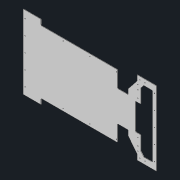
# Autodesk Inventor part: bellypanKJversion
Saved by Autodesk Inventor 2022 (Build 260153000, 153)
## iProperties
Created: 2022-09-22
Part Number: bellypanKJversion
Material: Generic
Document SubType Name: Modeling
Designer: Kieran Jarvis
Density: 1 g/cm^3
Appearance: Default
Author: Kieran Jarvis
Autodesk Inventor part; units mm, degrees
ref_plane "YZ Plane" through (0, 0, 0) normal (1, 0, 0) x (0, 1, 0)
ref_plane "XZ Plane" through (0, 0, 0) normal (0, 1, 0) x (-1, 0, 0)
ref_plane "XY Plane" through (0, 0, 0) normal (0, 0, 1) x (1, 0, 0)
sketch "Sketch1" plane through (0, 0, 0) normal (0, 0, 1) x (1, 0, 0)
  line L0 (0, 0) -> (0, 600) projected
  line L1 (900, 0) -> (900, 600) projected
  circle A0 centre (630, 497.5) radius 2.5 projected
  circle A1 centre (630, 102.5) radius 2.5 projected
  circle A2 centre (450, 102.5) radius 2.5 projected
  circle A3 centre (270, 102.5) radius 2.5 projected
  circle A4 centre (270, 497.5) radius 2.5 projected
  circle A5 centre (450, 497.5) radius 2.5 projected
  circle A6 centre (887.5, 500) radius 2.5 projected
  circle A7 centre (887.5, 400) radius 2.5 projected
  circle A8 centre (887.5, 300) radius 2.5 projected
  circle A9 centre (887.5, 200) radius 2.5 projected
  circle A10 centre (887.5, 100) radius 2.5 projected
  circle A11 centre (12.5, 500) radius 2.5 projected
  circle A12 centre (12.5, 400) radius 2.5 projected
  circle A13 centre (12.5, 300) radius 2.5 projected
  circle A14 centre (12.5, 200) radius 2.5 projected
  circle A15 centre (12.5, 100) radius 2.5 projected
  line L2 (875, 550) -> (25, 550) projected
  line L3 (875, 50) -> (25, 50) projected
  line L4 (875, 550) -> (900, 550)
  line L5 (875, 50) -> (900, 50)
  line L6 (25, 550) -> (0, 550)
  line L7 (25, 50) -> (0, 50)
  line L8 (875, 0) -> (875, 600) construction
  line L9 (795, 510) -> (795, 90) construction
  line L10 (875, 510) -> (25, 510) construction
  line L11 (875, 90) -> (25, 90) construction
  line L12 (875, 510) -> (875, 90)
  line L13 (875, 90) -> (815, 90)
  line L14 (815, 90) -> (815, 115)
  line L15 (815, 115) -> (795, 115)
  line L16 (875, 510) -> (815, 510)
  line L17 (815, 510) -> (815, 485)
  line L18 (815, 485) -> (795, 485)
  line L19 (763, 390) -> (787, 390) construction
  line L20 (787, 210) -> (763, 210) construction
  line L21 (795, 485) -> (795, 390)
  line L22 (758, 510) -> (758, 385) construction
  line L23 (758, 215) -> (758, 90) construction
  line L24 (795, 390) -> (758, 390)
  line L25 (795, 115) -> (795, 210)
  line L26 (795, 210) -> (758, 210)
  line L27 (758, 390) -> (758, 210)
  line L28 (780, 53) -> (780, 87) construction
  line L29 (780, 547) -> (780, 513) construction
  line L30 (780, 50) -> (770, 50) construction
  line L31 (770, 50) -> (770, 90) construction
  line L32 (770, 90) -> (780, 90) construction
  line L33 (780, 90) -> (780, 50) construction
  line L34 (780, 87) -> (120, 87) construction
  line L35 (780, 513) -> (120, 513) construction
  line L36 (770, 50) -> (770, 87)
  line L37 (770, 87) -> (120, 87)
  line L38 (120, 87) -> (120, 53) construction
  line L39 (120, 87) -> (120, 50)
  line L40 (780, 550) -> (770, 550) construction
  line L41 (770, 550) -> (770, 513) construction
  line L42 (770, 513) -> (780, 513) construction
  line L43 (780, 513) -> (780, 550) construction
  line L44 (770, 550) -> (770, 513)
  line L45 (770, 513) -> (120, 513)
  line L46 (120, 513) -> (120, 550)
  line L47 (795, 115) -> (815, 90)
  line L48 (815, 510) -> (795, 485)
  circle A16 centre (823.5, 530) radius 3 projected
  circle A17 centre (788.5, 530) radius 3 projected
  circle A18 centre (823.5, 70) radius 3 projected
  circle A19 centre (788.5, 70) radius 3 projected
  circle A20 centre (823.5, 70) radius 2.5
  circle A21 centre (788.5, 70) radius 2.5
  circle A22 centre (823.5, 530) radius 2.5
  circle A23 centre (788.5, 530) radius 2.5
  dimension "d0" = 60
  dimension "d1" = 25
  dimension "d2" = 60
  dimension "d3" = 25
  dimension "d4" = 10
  dimension "d5" = 10
  dimension "d37" = 5
  dimension "d38" = 5
  dimension "d39" = 5
  constraints: 64 end point, 29 point on line, 8 perpendicular, 6 parallel, 4 centre point, 4 coincident, 2 collinear, 2 horizontal, 2 vertical, 1 equal radius
  measures "d0" distance of L11.start L13.end
  measures "d1" distance of L13.end L14.end
  measures "d2" distance of L10.start L16.end
  measures "d3" distance of L16.end L17.end
  measures "d4" distance of L31.end L32.end
  measures "d5" distance of L42.end L41.end
  measures "d37" diameter of A20
  measures "d38" diameter of A22
  measures "d39" diameter of A23
extrude "Extrusion1" add sketch "Sketch1" along normal blind 3 contours L0 L6 L2 L46 L45 L44 L4 L1 L5 L3 L36 L37 L39 L7 | A16 | A17 | A18 | A19
fillet "Fillet1" radius 5 14 edges at (875, 90, 1.5) (815, 90, 1.5) (795, 115, 1.5) (795, 210, 1.5) (758, 210, 1.5) (758, 390, 1.5) (795, 390, 1.5) (795, 485, 1.5) (815, 510, 1.5) (875, 510, 1.5) (770, 87, 1.5) (120, 87, 1.5) (120, 513, 1.5) (770, 513, 1.5)
sketch "Sketch2" plane through (0, 0, 0) normal (0, 0, -1) x (-1, 0, 0)
  circle A0 centre (-12.5, 100) radius 2.5 projected
  circle A1 centre (-12.5, 300) radius 2.5 projected
  circle A2 centre (-12.5, 500) radius 2.5 projected
  circle A3 centre (-887.5, 200) radius 2.5 projected
  circle A4 centre (-887.5, 400) radius 2.5 projected
  circle A5 centre (-450, 497.5) radius 2.5 projected
  circle A6 centre (-270, 497.5) radius 2.5 projected
  circle A7 centre (-270, 102.5) radius 2.5 projected
  circle A8 centre (-450, 102.5) radius 2.5 projected
  circle A9 centre (-630, 102.5) radius 2.5 projected
  circle A10 centre (-630, 497.5) radius 2.5 projected
  circle A11 centre (-887.5, 500) radius 2.5 projected
  circle A12 centre (-887.5, 300) radius 2.5 projected
  circle A13 centre (-887.5, 100) radius 2.5 projected
  circle A14 centre (-12.5, 400) radius 2.5 projected
  circle A15 centre (-12.5, 200) radius 2.5 projected
  arc A16 (-765, 87) -> (-770, 82) centre (-765, 82) ccw projected
  line L0 (-125, 87) -> (-765, 87) projected
  arc A17 (-120, 82) -> (-125, 87) centre (-125, 82) ccw projected
  line L1 (-120, 50) -> (-120, 82) projected
  line L2 (0, 50) -> (-120, 50) projected
  line L3 (0, 550) -> (0, 50) projected
  line L4 (-120, 550) -> (0, 550) projected
  line L5 (-120, 518) -> (-120, 550) projected
  arc A18 (-125, 513) -> (-120, 518) centre (-125, 518) ccw projected
  line L6 (-765, 513) -> (-125, 513) projected
  arc A19 (-770, 518) -> (-765, 513) centre (-765, 518) ccw projected
  line L7 (-770, 550) -> (-770, 518) projected
  line L8 (-900, 550) -> (-770, 550) projected
  line L9 (-900, 50) -> (-900, 550) projected
  line L10 (-770, 50) -> (-900, 50) projected
  line L11 (-770, 82) -> (-770, 50) projected
  arc A20 (-795, 395) -> (-790, 390) centre (-790, 395) ccw projected
  line L12 (-763, 390) -> (-790, 390) projected
  arc A21 (-758, 385) -> (-763, 390) centre (-763, 385) ccw projected
  line L13 (-758, 215) -> (-758, 385) projected
  arc A22 (-763, 210) -> (-758, 215) centre (-763, 215) ccw projected
  line L14 (-790, 210) -> (-763, 210) projected
  arc A23 (-790, 210) -> (-795, 205) centre (-790, 205) ccw projected
  line L15 (-795, 116.7539) -> (-795, 205) projected
  arc A24 (-796.0957, 113.6304) -> (-795, 116.7539) centre (-800, 116.7539) ccw projected
  line L16 (-813.4988, 91.8765) -> (-796.0957, 113.6304) projected
  arc A25 (-817.4031, 90) -> (-813.4988, 91.8765) centre (-817.4031, 95) ccw projected
  line L17 (-870, 90) -> (-817.4031, 90) projected
  arc A26 (-875, 95) -> (-870, 90) centre (-870, 95) ccw projected
  line L18 (-875, 505) -> (-875, 95) projected
  arc A27 (-870, 510) -> (-875, 505) centre (-870, 505) ccw projected
  line L19 (-817.4031, 510) -> (-870, 510) projected
  arc A28 (-813.4988, 508.1235) -> (-817.4031, 510) centre (-817.4031, 505) ccw projected
  line L20 (-796.0957, 486.3696) -> (-813.4988, 508.1235) projected
  arc A29 (-795, 483.2461) -> (-796.0957, 486.3696) centre (-800, 483.2461) ccw projected
  line L21 (-795, 395) -> (-795, 483.2461) projected
  line L22 (-125, 87) -> (-765, 87) construction
  line L23 (-770, 50) -> (-735, 50) construction
  line L24 (-735, 50) -> (-735, 87) construction
  line L25 (-735, 87) -> (-770, 87) construction
  line L26 (-770, 87) -> (-770, 50) construction
  line L27 (-735, 50) -> (-637, 50) construction
  line L28 (-637, 50) -> (-637, 87) construction
  line L29 (-637, 87) -> (-735, 87) construction
  line L30 (-735, 87) -> (-735, 50) construction
  line L31 (-735, 87) -> (-735, 122)
  line L32 (-735, 122) -> (-710, 122)
  line L33 (-710, 122) -> (-710, 197)
  line L34 (-637, 87) -> (-637, 197)
  line L35 (-637, 197) -> (-710, 197)
  line L36 (-758, 215) -> (-758, 385) construction
  line L37 (-758, 300) -> (0, 300) construction
  line L38 (0, 550) -> (0, 50) construction
  line L39 (-735, 513) -> (-735, 478)
  line L40 (-735, 478) -> (-710, 478)
  line L41 (-710, 478) -> (-710, 403)
  line L42 (-637, 513) -> (-637, 403)
  line L43 (-637, 403) -> (-710, 403)
  point P0 (0, 0)
  point P1 (-637, 513)
  point P2 (-735, 513)
  point P3 (-735, 87)
  point P4 (-637, 87)
  dimension "d9" = 35
  dimension "d10" = 98
  dimension "d11" = 35
  dimension "d12" = 25
  dimension "d13" = 75
  constraints: 38 end point, 6 symmetric about line, 5 perpendicular, 4 parallel, 3 point on line, 2 horizontal, 2 midpoint, 1 vertical
  measures "d9" distance of L25.end L24.end
  measures "d10" distance of L29.end L28.end
  measures "d11" distance of L29.end L31.end
  measures "d12" distance of L31.end L32.end
  measures "d13" distance of L32.end L33.end
extrude "Extrusion2" cut sketch "Sketch2" against normal blind 3 contours L31 L32 L33 L35 L34 L0 | L6 L42 L43 L41 L40 L39
fillet "Fillet2" radius 5 10 edges at (735, 87, 1.5) (735, 122, 1.5) (710, 122, 1.5) (710, 197, 1.5) (637, 197, 1.5) (637, 87, 1.5) (637, 403, 1.5) (710, 403, 1.5) (710, 478, 1.5) (735, 478, 1.5)
sketch "Sketch3" plane through (0, 0, 3) normal (0, 0, 1) x (1, 0, 0)
  arc A0 (715, 478) -> (710, 473) centre (715, 473) ccw projected
  line L0 (710, 473) -> (710, 408) projected
  arc A1 (705, 403) -> (710, 408) centre (705, 408) ccw projected
  line L1 (705, 403) -> (642, 403) projected
  arc A2 (637, 408) -> (642, 403) centre (642, 408) ccw projected
  line L2 (637, 408) -> (637, 513) projected
  line L3 (637, 513) -> (125, 513) projected
  arc A3 (120, 518) -> (125, 513) centre (125, 518) ccw projected
  line L4 (120, 518) -> (120, 550) projected
  line L5 (120, 550) -> (0, 550) projected
  line L6 (0, 550) -> (0, 50) projected
  line L7 (0, 50) -> (120, 50) projected
  line L8 (120, 50) -> (120, 82) projected
  arc A4 (125, 87) -> (120, 82) centre (125, 82) ccw projected
  line L9 (125, 87) -> (632, 87) projected
  arc A5 (632, 87) -> (637, 92) centre (632, 92) ccw projected
  line L10 (637, 92) -> (637, 192) projected
  arc A6 (642, 197) -> (637, 192) centre (642, 192) ccw projected
  line L11 (642, 197) -> (705, 197) projected
  arc A7 (710, 192) -> (705, 197) centre (705, 192) ccw projected
  line L12 (710, 192) -> (710, 127) projected
  arc A8 (710, 127) -> (715, 122) centre (715, 127) ccw projected
  line L13 (715, 122) -> (730, 122) projected
  arc A9 (735, 117) -> (730, 122) centre (730, 117) ccw projected
  line L14 (735, 117) -> (735, 92) projected
  arc A10 (735, 92) -> (740, 87) centre (740, 92) ccw projected
  line L15 (740, 87) -> (765, 87) projected
  arc A11 (770, 82) -> (765, 87) centre (765, 82) ccw projected
  line L16 (770, 82) -> (770, 50) projected
  line L17 (770, 50) -> (900, 50) projected
  line L18 (900, 50) -> (900, 550) projected
  line L19 (900, 550) -> (770, 550) projected
  line L20 (770, 550) -> (770, 518) projected
  arc A12 (765, 513) -> (770, 518) centre (765, 518) ccw projected
  line L21 (765, 513) -> (735, 513) projected
  line L22 (735, 513) -> (735, 483) projected
  arc A13 (730, 478) -> (735, 483) centre (730, 483) ccw projected
  line L23 (730, 478) -> (715, 478) projected
  circle A14 centre (12.5, 200) radius 2.5 projected
  circle A15 centre (12.5, 400) radius 2.5 projected
  circle A16 centre (887.5, 100) radius 2.5 projected
  circle A17 centre (887.5, 300) radius 2.5 projected
  circle A18 centre (887.5, 500) radius 2.5 projected
  circle A19 centre (630, 497.5) radius 2.5 projected
  circle A20 centre (630, 102.5) radius 2.5 projected
  circle A21 centre (450, 102.5) radius 2.5 projected
  circle A22 centre (270, 102.5) radius 2.5 projected
  circle A23 centre (270, 497.5) radius 2.5 projected
  circle A24 centre (450, 497.5) radius 2.5 projected
  circle A25 centre (887.5, 400) radius 2.5 projected
  circle A26 centre (887.5, 200) radius 2.5 projected
  circle A27 centre (12.5, 500) radius 2.5 projected
  circle A28 centre (12.5, 300) radius 2.5 projected
  circle A29 centre (12.5, 100) radius 2.5 projected
  arc A30 (790, 390) -> (795, 395) centre (790, 395) ccw projected
  line L24 (795, 395) -> (795, 483.2461) projected
  arc A31 (796.0957, 486.3696) -> (795, 483.2461) centre (800, 483.2461) ccw projected
  line L25 (796.0957, 486.3696) -> (813.4988, 508.1235) projected
  arc A32 (817.4031, 510) -> (813.4988, 508.1235) centre (817.4031, 505) ccw projected
  line L26 (817.4031, 510) -> (870, 510) projected
  arc A33 (875, 505) -> (870, 510) centre (870, 505) ccw projected
  line L27 (875, 505) -> (875, 95) projected
  arc A34 (870, 90) -> (875, 95) centre (870, 95) ccw projected
  line L28 (870, 90) -> (817.4031, 90) projected
  arc A35 (813.4988, 91.8765) -> (817.4031, 90) centre (817.4031, 95) ccw projected
  line L29 (813.4988, 91.8765) -> (796.0957, 113.6304) projected
  arc A36 (795, 116.7539) -> (796.0957, 113.6304) centre (800, 116.7539) ccw projected
  line L30 (795, 116.7539) -> (795, 205) projected
  arc A37 (795, 205) -> (790, 210) centre (790, 205) ccw projected
  line L31 (790, 210) -> (763, 210) projected
  arc A38 (758, 215) -> (763, 210) centre (763, 215) ccw projected
  line L32 (758, 215) -> (758, 385) projected
  arc A39 (763, 390) -> (758, 385) centre (763, 385) ccw projected
  line L33 (763, 390) -> (790, 390) projected
  line L34 (795, 510) -> (795, 90) projected
  line L35 (763, 390) -> (790, 390) construction
  line L36 (795, 510) -> (775, 510) construction
  line L37 (775, 510) -> (775, 390) construction
  line L38 (775, 390) -> (795, 390) construction
  line L39 (795, 390) -> (795, 510) construction
  line L40 (795, 510) -> (775, 510) construction
  line L41 (775, 510) -> (775, 465) construction
  line L42 (775, 465) -> (795, 465) construction
  line L43 (795, 465) -> (795, 510) construction
  line L44 (795, 510) -> (775, 510) construction
  line L45 (775, 510) -> (775, 495) construction
  line L46 (775, 495) -> (795, 495) construction
  line L47 (795, 495) -> (795, 510) construction
  line L48 (795, 90) -> (775, 90) construction
  line L49 (775, 90) -> (775, 135) construction
  line L50 (775, 135) -> (795, 135) construction
  line L51 (795, 135) -> (795, 90) construction
  line L52 (795, 90) -> (775, 90) construction
  line L53 (775, 90) -> (775, 105) construction
  line L54 (775, 105) -> (795, 105) construction
  line L55 (795, 105) -> (795, 90) construction
  circle A40 centre (775, 105) radius 2.5 projected
  circle A41 centre (775, 135) radius 2.5 projected
  line L56 (775, 135) -> (795.2819, 135) construction
  line L57 (795.2819, 135) -> (795.2819, 185) construction
  line L58 (795.2819, 185) -> (775, 185) construction
  line L59 (775, 185) -> (775, 135) construction
  line L60 (795, 465) -> (775, 465) construction
  line L61 (775, 465) -> (775, 415) construction
  line L62 (775, 415) -> (795, 415) construction
  line L63 (795, 415) -> (795, 465) construction
  point P0 (0, 0)
  dimension "d17" = 20
  dimension "d18" = 45
  dimension "d19" = 15
  dimension "d20" = 20
  dimension "d21" = 45
  dimension "d22" = 20
  dimension "d23" = 15
  dimension "d31" = 50
  dimension "d32" = 50
  constraints: 56 end point, 14 parallel, 7 horizontal, 7 perpendicular, 6 coincident, 4 point on line
  measures "d17" distance of L38.end L37.end
  measures "d18" distance of L41.end L40.end
  measures "d19" distance of L45.end L44.end
  measures "d20" distance of L49.end L50.end
  measures "d21" distance of L48.end L49.end
  measures "d22" distance of L53.end L54.end
  measures "d23" distance of L52.end L53.end
  measures "d31" distance of L57.end L56.end
  measures "d32" distance of L61.end L60.end
hole "Hole1" at (775, 465, 3) at (775, 495, 3) at (775, 135, 3) at (775, 105, 3) at (775, 415, 3) at (775, 185, 3) direction (0, 0, -1) diameter 5 depth 8 tip angle 118
sketch "Sketch4" plane through (0, 0, 3) normal (0, 0, 1) x (1, 0, 0)
  circle A0 centre (775, 415) radius 2.5 projected
  circle A1 centre (775, 135) radius 2.5 projected
  circle A2 centre (775, 465) radius 2.5 projected
  circle A3 centre (775, 495) radius 2.5 projected
  circle A4 centre (775, 105) radius 2.5 projected
  circle A5 centre (775, 185) radius 2.5 projected
  arc A6 (715, 478) -> (710, 473) centre (715, 473) ccw projected
  line L0 (710, 473) -> (710, 408) projected
  arc A7 (705, 403) -> (710, 408) centre (705, 408) ccw projected
  line L1 (705, 403) -> (642, 403) projected
  arc A8 (637, 408) -> (642, 403) centre (642, 408) ccw projected
  line L2 (637, 408) -> (637, 513) projected
  line L3 (637, 513) -> (125, 513) projected
  arc A9 (120, 518) -> (125, 513) centre (125, 518) ccw projected
  line L4 (120, 518) -> (120, 550) projected
  line L5 (120, 550) -> (0, 550) projected
  line L6 (0, 550) -> (0, 50) projected
  line L7 (0, 50) -> (120, 50) projected
  line L8 (120, 50) -> (120, 82) projected
  arc A10 (125, 87) -> (120, 82) centre (125, 82) ccw projected
  line L9 (125, 87) -> (632, 87) projected
  arc A11 (632, 87) -> (637, 92) centre (632, 92) ccw projected
  line L10 (637, 92) -> (637, 192) projected
  arc A12 (642, 197) -> (637, 192) centre (642, 192) ccw projected
  line L11 (642, 197) -> (705, 197) projected
  arc A13 (710, 192) -> (705, 197) centre (705, 192) ccw projected
  line L12 (710, 192) -> (710, 127) projected
  arc A14 (710, 127) -> (715, 122) centre (715, 127) ccw projected
  line L13 (715, 122) -> (730, 122) projected
  arc A15 (735, 117) -> (730, 122) centre (730, 117) ccw projected
  line L14 (735, 117) -> (735, 92) projected
  arc A16 (735, 92) -> (740, 87) centre (740, 92) ccw projected
  line L15 (740, 87) -> (765, 87) projected
  arc A17 (770, 82) -> (765, 87) centre (765, 82) ccw projected
  line L16 (770, 82) -> (770, 50) projected
  line L17 (770, 50) -> (900, 50) projected
  line L18 (900, 50) -> (900, 550) projected
  line L19 (900, 550) -> (770, 550) projected
  line L20 (770, 550) -> (770, 518) projected
  arc A18 (765, 513) -> (770, 518) centre (765, 518) ccw projected
  line L21 (765, 513) -> (735, 513) projected
  line L22 (735, 513) -> (735, 483) projected
  arc A19 (730, 478) -> (735, 483) centre (730, 483) ccw projected
  line L23 (730, 478) -> (715, 478) projected
  circle A20 centre (12.5, 200) radius 2.5 projected
  circle A21 centre (12.5, 400) radius 2.5 projected
  circle A22 centre (887.5, 100) radius 2.5 projected
  circle A23 centre (887.5, 300) radius 2.5 projected
  circle A24 centre (887.5, 500) radius 2.5 projected
  circle A25 centre (630, 497.5) radius 2.5 projected
  circle A26 centre (630, 102.5) radius 2.5 projected
  circle A27 centre (450, 102.5) radius 2.5 projected
  circle A28 centre (270, 102.5) radius 2.5 projected
  circle A29 centre (270, 497.5) radius 2.5 projected
  circle A30 centre (450, 497.5) radius 2.5 projected
  circle A31 centre (887.5, 400) radius 2.5 projected
  circle A32 centre (887.5, 200) radius 2.5 projected
  circle A33 centre (12.5, 500) radius 2.5 projected
  circle A34 centre (12.5, 300) radius 2.5 projected
  circle A35 centre (12.5, 100) radius 2.5 projected
  arc A36 (790, 390) -> (795, 395) centre (790, 395) ccw projected
  line L24 (795, 395) -> (795, 483.2461) projected
  arc A37 (796.0957, 486.3696) -> (795, 483.2461) centre (800, 483.2461) ccw projected
  line L25 (796.0957, 486.3696) -> (813.4988, 508.1235) projected
  arc A38 (817.4031, 510) -> (813.4988, 508.1235) centre (817.4031, 505) ccw projected
  line L26 (817.4031, 510) -> (870, 510) projected
  arc A39 (875, 505) -> (870, 510) centre (870, 505) ccw projected
  line L27 (875, 505) -> (875, 95) projected
  arc A40 (870, 90) -> (875, 95) centre (870, 95) ccw projected
  line L28 (870, 90) -> (817.4031, 90) projected
  arc A41 (813.4988, 91.8765) -> (817.4031, 90) centre (817.4031, 95) ccw projected
  line L29 (813.4988, 91.8765) -> (796.0957, 113.6304) projected
  arc A42 (795, 116.7539) -> (796.0957, 113.6304) centre (800, 116.7539) ccw projected
  line L30 (795, 116.7539) -> (795, 205) projected
  arc A43 (795, 205) -> (790, 210) centre (790, 205) ccw projected
  line L31 (790, 210) -> (763, 210) projected
  arc A44 (758, 215) -> (763, 210) centre (763, 215) ccw projected
  line L32 (758, 215) -> (758, 385) projected
  arc A45 (763, 390) -> (758, 385) centre (763, 385) ccw projected
  line L33 (763, 390) -> (790, 390) projected
  line L34 (770, 87) -> (710, 162)
  line L35 (813.4988, 91.8765) -> (796.0957, 113.6304) projected
  arc A46 (770, 82) -> (765, 87) centre (765, 82) ccw projected
  line L36 (770, 82) -> (770, 87)
  line L37 (770, 82) -> (770, 50) projected
  line L38 (770, 87) -> (765, 87)
  line L39 (758, 215) -> (758, 385) projected
  line L40 (758, 300) -> (660.4411, 300)
  line L41 (758, 300) -> (855.5589, 300) construction
  line L42 (770, 513) -> (710, 438)
  line L43 (770, 518) -> (770, 513)
  line L44 (770, 513) -> (765, 513)
  point P0 (0, 0)
  dimension "d36" = 180
  constraints: 16 end point, 2 collinear, 2 symmetric about line, 1 horizontal, 1 midpoint, 1 parallel, 1 perpendicular, 1 point on line, 1 tangent
  measures "d36" angle of L40 L41
extrude "Extrusion3" cut sketch "Sketch4" against normal blind 3 contours L23 A19 L22 L21 L44 L42 L0 A6 | L44 A18 L43 | A17 L38 L36 | L15 A16 L14 A15 L13 A14 L12 L34 L38
fillet "Fillet3" radius 5 4 edges at (710, 162, 1.5) (770, 87, 1.5) (710, 438, 1.5) (770, 513, 1.5)
body "Solid1"
